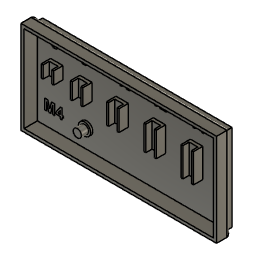
M4 Reference Caliper From 6 v4 (Autodesk Fusion 360 design; units mm, degrees)
Autodesk Fusion 360 part; units mm, degrees
note: some values were not read from the file. Chosen so that the rebuilt part matches the saved one: which bodies a step acts on; which pieces of a blend or face edit are solid.
sketch "Schizzo1" plane through (0, 0, 0) normal (0, 1, 0) x (1, 0, 0)
  line L0 (-43.0702, -47.1256) -> (51.9298, -47.1256)
  line L1 (51.9298, -47.1256) -> (51.9298, -2.1256)
  line L2 (51.9298, -2.1256) -> (-43.0702, -2.1256)
  line L3 (-43.0702, -2.1256) -> (-43.0702, -47.1256)
  line L4 (-34.9398, -37.9923) -> (-30.6504, -37.9923) construction
  line L5 (-30.6504, -37.9923) -> (-30.6504, -43.6096) construction
  line L6 (-30.6504, -43.6096) -> (-34.9398, -43.6096) construction
  line L7 (-34.9398, -43.6096) -> (-34.9398, -37.9923) construction
  line L8 (-20.4362, -37.9923) -> (-16.447, -37.9923) construction
  line L9 (-16.447, -37.9923) -> (-16.447, -43.6096) construction
  line L10 (-16.447, -43.6096) -> (-20.4362, -43.6096) construction
  line L11 (-20.4362, -43.6096) -> (-20.4362, -37.9923) construction
  line L12 (-2.7087, -37.9923) -> (2.1333, -37.9923) construction
  line L13 (2.1333, -37.9923) -> (2.1333, -43.6096) construction
  line L14 (2.1333, -43.6096) -> (-2.7087, -43.6096) construction
  line L15 (-2.7087, -43.6096) -> (-2.7087, -37.9923) construction
  line L16 (14.1885, -37.9923) -> (20.8281, -37.9923) construction
  line L17 (20.8281, -37.9923) -> (20.8281, -43.6096) construction
  line L18 (20.8281, -43.6096) -> (14.1885, -43.6096) construction
  line L19 (14.1885, -43.6096) -> (14.1885, -37.9923) construction
  line L20 (32.7115, -37.9923) -> (40.1532, -37.9923) construction
  line L21 (40.1532, -37.9923) -> (40.1532, -43.6096) construction
  line L22 (40.1532, -43.6096) -> (32.7115, -43.6096) construction
  line L23 (32.7115, -43.6096) -> (32.7115, -37.9923) construction
  line L24 (-35.1629, -33.0713) -> (-29.1629, -33.0713)
  line L25 (-29.1629, -33.0713) -> (-29.1629, -27.0713)
  line L26 (-29.1629, -27.0713) -> (-35.1629, -27.0713)
  line L27 (-35.1629, -27.0713) -> (-35.1629, -33.0713)
  line L28 (-32.1629, -33.0713) -> (-32.1629, -27.0713) construction
  line L29 (-30.0629, -27.0713) -> (-34.2629, -27.0713)
  line L30 (-34.2629, -27.0713) -> (-34.2629, -33.0713)
  line L31 (-34.2629, -33.0713) -> (-30.0629, -33.0713)
  line L32 (-30.0629, -33.0713) -> (-30.0629, -27.0713)
  line L33 (-30.0629, -27.0713) -> (-34.2629, -33.0713) construction
  line L34 (-34.2629, -27.0713) -> (-30.0629, -33.0713) construction
  line L35 (-14.9964, -25.0713) -> (-20.9964, -25.0713)
  line L36 (-20.0964, -25.0713) -> (-15.8964, -33.0713) construction
  line L37 (-15.8964, -25.0713) -> (-20.0964, -25.0713)
  line L38 (-15.8964, -33.0713) -> (-15.8964, -25.0713)
  line L39 (-20.0964, -25.0713) -> (-20.0964, -33.0713)
  line L40 (-15.8964, -25.0713) -> (-20.0964, -33.0713) construction
  line L41 (-17.9964, -33.0713) -> (-17.9964, -25.0713) construction
  line L42 (-20.9964, -33.0713) -> (-14.9964, -33.0713)
  line L43 (-20.9964, -25.0713) -> (-20.9964, -33.0713)
  line L44 (-14.9964, -33.0713) -> (-14.9964, -25.0713)
  line L45 (-20.0964, -33.0713) -> (-15.8964, -33.0713)
  line L46 (1.6974, -33.0713) -> (1.6974, -23.0713)
  line L47 (-3.4026, -23.0713) -> (-3.4026, -33.0713)
  line L48 (2.5974, -33.0713) -> (2.5974, -23.0713)
  line L49 (-3.4026, -33.0713) -> (2.5974, -33.0713)
  line L50 (1.6974, -23.0713) -> (-2.5026, -33.0713) construction
  line L51 (1.6974, -23.0713) -> (-2.5026, -23.0713)
  line L52 (-2.5026, -23.0713) -> (-2.5026, -33.0713)
  line L53 (-2.5026, -23.0713) -> (1.6974, -33.0713) construction
  line L54 (2.5974, -23.0713) -> (-3.4026, -23.0713)
  line L55 (-0.4026, -33.0713) -> (-0.4026, -23.0713) construction
  line L56 (-2.5026, -33.0713) -> (1.6974, -33.0713)
  line L57 (15.58, -33.0713) -> (19.78, -33.0713)
  line L58 (15.58, -21.0713) -> (15.58, -33.0713)
  line L59 (14.68, -33.0713) -> (20.68, -33.0713)
  line L60 (19.78, -33.0713) -> (19.78, -21.0713)
  line L61 (19.78, -21.0713) -> (15.58, -33.0713) construction
  line L62 (20.68, -21.0713) -> (14.68, -21.0713)
  line L63 (17.68, -33.0713) -> (17.68, -21.0713) construction
  line L64 (14.68, -21.0713) -> (14.68, -33.0713)
  line L65 (19.78, -21.0713) -> (15.58, -21.0713)
  line L66 (15.58, -21.0713) -> (19.78, -33.0713) construction
  line L67 (20.68, -33.0713) -> (20.68, -21.0713)
  line L68 (-43.0702, -33.0713) -> (51.9298, -33.0713) construction
  line L69 (32.7212, -33.0713) -> (38.7212, -33.0713)
  line L70 (37.8212, -19.0713) -> (33.6212, -33.0713) construction
  line L71 (38.7212, -33.0713) -> (38.7212, -19.0713)
  line L72 (32.7212, -19.0713) -> (32.7212, -33.0713)
  line L73 (37.8212, -33.0713) -> (37.8212, -19.0713)
  line L74 (37.8212, -19.0713) -> (33.6212, -19.0713)
  line L75 (35.7212, -33.0713) -> (35.7212, -19.0713) construction
  line L76 (33.6212, -19.0713) -> (33.6212, -33.0713)
  line L77 (33.6212, -33.0713) -> (37.8212, -33.0713)
  line L78 (33.6212, -19.0713) -> (37.8212, -33.0713) construction
  line L79 (38.7212, -19.0713) -> (32.7212, -19.0713)
  line L80 (-43.0702, -43.6096) -> (51.9298, -43.6096) construction
  line L81 (50.4298, -45.6256) -> (50.4298, -3.6256)
  line L82 (50.4298, -3.6256) -> (-41.5702, -3.6256)
  line L83 (-41.5702, -3.6256) -> (-41.5702, -45.6256)
  line L84 (-41.5702, -45.6256) -> (50.4298, -45.6256)
  line L85 (-38, -10) -> (-25, -10) construction
  line L86 (-25, -10) -> (-25, -15) construction
  line L87 (-25, -15) -> (-38, -15) construction
  line L88 (-38, -15) -> (-38, -10) construction
  line L89 (-43.0702, -37.9923) -> (50.4298, -37.9923) construction
  circle A0 centre (-17.6815, -12.6421) radius 2
  circle A1 centre (-17.6815, -12.6421) radius 3
  point P0 (-32.1629, -30.0713)
  point P1 (-17.9964, -29.0713)
  point P2 (-0.4026, -28.0713)
  point P3 (17.68, -27.0713)
  point P4 (35.7212, -26.0713)
  dimension "d1" = 45
  dimension "d2" = 5
  dimension "d3" = 5
  dimension "d4" = 5
  dimension "d5" = 5
  dimension "d6" = 5
  dimension "d7" = 6
  dimension "d8" = 6
  dimension "d9" = 4.2
  dimension "d21" = 6
  dimension "d22" = 8
  dimension "d23" = 4.2
  dimension "d24" = 6
  dimension "d25" = 10
  dimension "d26" = 4.2
  dimension "d27" = 6
  dimension "d28" = 12
  dimension "d29" = 4.2
  dimension "d30" = 6
  dimension "d31" = 14
  dimension "d32" = 4.2
  dimension "d33" = 95
  dimension "d34" = -1.5
  dimension "d37" = 5
  dimension "d40" = 4
  dimension "d41" = 6
  text T0 "6" font "Arial" height 5 bold align left middle in box 4.2894 x 5.6173 at (-34.9398, -37.9923) x (1, 0) y (0, -1) spacing 1
  text T1 "8" font "Arial" height 5 bold align left top in box 3.9891 x 5.6173 at (-20.4362, -37.9923) x (1, 0) y (0, -1) spacing 1
  text T2 "10\n" font "Arial" height 5 bold align left top in box 4.842 x 5.6173 at (-2.7087, -37.9923) x (1, 0) y (0, -1) spacing 1
  text T3 "12" font "Arial" height 5 bold align left top in box 6.6397 x 5.6173 at (14.1885, -37.9923) x (1, 0) y (0, -1) spacing 1
  text T4 "14" font "Arial" height 5 bold align left top in box 7.4417 x 5.6173 at (32.7115, -37.9923) x (1, 0) y (0, -1) spacing 1
  text T5 "M4" font "Arial" height 5 bold align left top in box 13 x 5 at (-38, -10) x (1, 0) y (0, -1) spacing 1
  constraint horizontal L0
  constraint vertical L1
  constraint horizontal L2
  constraint vertical L3
  constraint horizontal L24
  constraint vertical L25
  constraint horizontal L26
  constraint vertical L27
  constraint midpoint L24 L28.start
  constraint midpoint L26 L28.end
  constraint horizontal L29
  constraint perpendicular L29 L30
  constraint parallel L29 L31
  constraint parallel L30 L32
  constraint coincident L33 P0
  constraint coincident L34 P0
  constraint coincident L26 L29.start
  constraint midpoint L28 P0
  constraint horizontal L42
  constraint vertical L44
  constraint horizontal L35
  constraint vertical L43
  constraint midpoint L41.start L42
  constraint midpoint L41.end L35
  constraint horizontal L37
  constraint perpendicular L37 L39
  constraint parallel L37 L45
  constraint parallel L38 L39
  constraint coincident P1 L40
  constraint coincident P1 L36
  constraint coincident L37.start L35
  constraint midpoint P1 L41
  constraint horizontal L49
  constraint vertical L48
  constraint horizontal L54
  constraint vertical L47
  constraint midpoint L55.start L49
  constraint midpoint L55.end L54
  constraint horizontal L51
  constraint perpendicular L51 L52
  constraint parallel L51 L56
  constraint parallel L46 L52
  constraint coincident P2 L50
  constraint coincident P2 L53
  constraint coincident L46.end L54
  constraint midpoint P2 L55
  constraint horizontal L59
  constraint vertical L67
  constraint horizontal L62
  constraint vertical L64
  constraint midpoint L63.start L59
  constraint midpoint L63.end L62
  constraint horizontal L65
  constraint perpendicular L58 L65
  constraint parallel L57 L65
  constraint parallel L58 L60
  constraint coincident P3 L61
  constraint coincident P3 L66
  constraint coincident L60.end L62
  constraint midpoint P3 L63
  constraint coincident L3 L68.start
  constraint coincident L1 L68.end
  constraint perpendicular L1 L68
  constraint collinear L31 L68
  constraint collinear L49 L68
  constraint collinear L59 L68
  constraint horizontal L69
  constraint vertical L71
  constraint horizontal L79
  constraint vertical L72
  constraint midpoint L75.start L69
  constraint midpoint L75.end L79
  constraint horizontal L74
  constraint perpendicular L74 L76
  constraint parallel L74 L77
  constraint parallel L73 L76
  constraint coincident P4 L70
  constraint coincident P4 L78
  constraint coincident L70.start L79
  constraint midpoint P4 L75
  constraint coincident L3 L80.start
  constraint coincident L1 L80.end
  constraint perpendicular L1 L80
  constraint collinear L42 L68
  constraint collinear L68 L69
  constraint collinear L6 L80
  constraint collinear L10 L80
  constraint collinear L14 L80
  constraint collinear L18 L80
  constraint collinear L22 L80
  constraint coincident L3 L89.start
  constraint coincident L81 L89.end
  constraint perpendicular L81 L89
  constraint collinear L4 L89
  constraint collinear L8 L89
  constraint collinear L12 L89
  constraint collinear L16 L89
  constraint collinear L20 L89
  constraint concentric A0 A1
  measures "d1" distance of L0 L2
  measures "d7" distance of L24.start L24.end
  measures "d8" distance of L24.start L26.end
  measures "d9" distance of L30 L32
  measures "d21" distance of L42.start L42.end
  measures "d22" distance of L42.start L35.end
  measures "d23" distance of L38 L39
  measures "d24" distance of L47.end L48.start
  measures "d25" distance of L47.start L47.end
  measures "d26" distance of L46 L52
  measures "d27" distance of L59.end L59.start
  measures "d28" distance of L62.end L59.start
  measures "d29" distance of L58 L60
  measures "d30" distance of L69.start L69.end
  measures "d31" distance of L69.start L72.start
  measures "d32" distance of L73 L76
  measures "d33" distance of L1 L3
  measures "d40" diameter of A0
  measures "d41" diameter of A1
extrude "Estrusione1" add sketch "Schizzo1" along normal blind 0.4 text T0 T1 T2 T3 T4 T5 makes body 1 at (-34.2253, 0, 40.762) makes body 2 at (38.8382, 0, 42.0851) makes body 3 at (3.8192, 0, 40.7205) makes body 4 at (-18.3806, 0, 41.2901) makes body 5 at (19.2999, 0, 38.9063) makes body 6 at (34.5885, 0, 41.4871) makes body 7 at (-29.8815, 0, 13.4754) makes body 8 at (-37.6874, 0, 12.9786) makes body 9 at (-0.8317, 0, 41.4871) makes body 10 at (16.0655, 0, 41.4871)
extrude "Estrusione2" add sketch "Schizzo1" along normal blind 0.5 separate body contours L0 L1 L2 L3 | L24 L26 L27 L30 | L24 L26 L29 L30 L31 L32 | L24 L25 L26 L32 | L35 L38 L42 L44 | L35 L37 L38 L39 L42 L45 | L35 L39 L42 L43 | L46 L49 L51 L52 L54 L56 | L46 L48 L49 L54 | L47 L49 L52 L54 | L57 L58 L59 L60 L62 L65 | L58 L59 L62 L64 | L59 L60 L62 L67 | L69 L72 L76 L79 | L69 L73 L74 L76 L77 L79 | L69 L71 L73 L79 | L81 L82 L83 L84 | A0 | A1 makes body 11
extrude "Estrusione7" cut sketch "Schizzo1" along normal blind 0.4 text T0 T1 T2 T3 T5 T4 bodies 11
extrude "Estrusione6" add sketch "Schizzo1" against normal blind 6.5 contours L0 L1 L2 L3 bodies 11
extrude "Estrusione4" add sketch "Schizzo1" against normal blind 4.5 contours L24 L26 L27 L30 | L24 L26 L29 L30 L31 L32 | L24 L25 L26 L32 | L35 L38 L42 L44 | L35 L37 L38 L39 L42 L45 | L35 L39 L42 L43 | L46 L49 L51 L52 L54 L56 | L46 L48 L49 L54 | L47 L49 L52 L54 | L57 L58 L59 L60 L62 L65 | L58 L59 L62 L64 | L59 L60 L62 L67 | L69 L72 L76 L79 | L69 L73 L74 L76 L77 L79 | L69 L71 L73 L79 | A0 bodies 11
extrude "Estrusione8" add sketch "Schizzo1" against normal blind 1 contours A1 bodies 11
extrude "Estrusione5" cut sketch "Schizzo1" along normal blind 3 from surface at -4.5 contours L24 L26 L29 L30 L31 L32 | L35 L37 L38 L39 L42 L45 | L46 L49 L51 L52 L54 L56 | L57 L58 L59 L60 L62 L65 | L69 L73 L74 L76 L77 L79 bodies 11
sketch "Schizzo2" plane through (0, 0.5, 0) normal (0, 1, 0) x (-1, 0, 0)
  line L0 (43.0702, 2.1256) -> (43.0702, 47.1256)
  line L1 (43.0702, 47.1256) -> (-51.9298, 47.1256)
  line L2 (-51.9298, 47.1256) -> (-51.9298, 2.1256)
  line L3 (-51.9298, 2.1256) -> (43.0702, 2.1256)
  line L4 (-51.9298, 47.1256) -> (43.0702, 47.1256) construction
  line L5 (43.0702, 47.1256) -> (43.0702, 2.1256) construction
  line L6 (43.0702, 2.1256) -> (-51.9298, 2.1256) construction
  line L7 (-51.9298, 2.1256) -> (-51.9298, 47.1256) construction
  line L8 (-51.9298, 24.6256) -> (-50, 24.6256) construction
  line L9 (-50, 24.6256) -> (43.0702, 24.6256) construction
  line L10 (-4.4298, 47.1256) -> (-4.4298, 2.1256) construction
  line L11 (41.5702, 3.6256) -> (-50.4298, 3.6256)
  line L12 (-50.4298, 3.6256) -> (-50.4298, 45.6256)
  line L13 (-50.4298, 45.6256) -> (41.5702, 45.6256)
  line L14 (41.5702, 45.6256) -> (41.5702, 3.6256)
  line L15 (41.5702, 3.6256) -> (-50.4298, 45.6256) construction
  line L16 (-50.4298, 3.6256) -> (41.5702, 45.6256) construction
  point P0 (-4.4298, 24.6256)
  dimension "d44" = 1.5
  dimension "d45" = 1.5
  constraint horizontal L4
  constraint vertical L5
  constraint horizontal L6
  constraint vertical L7
  constraint coincident L0.end L1.start
  constraint coincident L2.end L3.start
  constraint midpoint L7 L8.start
  constraint perpendicular L7 L8
  constraint midpoint L5 L9.end
  constraint perpendicular L5 L9
  constraint midpoint L4 L10.start
  constraint midpoint L6 L10.end
  constraint horizontal L11
  constraint perpendicular L11 L12
  constraint parallel L11 L13
  constraint parallel L12 L14
  constraint coincident L15 P0
  constraint coincident L16 P0
  constraint midpoint L10 P0
  measures "d44" distance of L7 L12
  measures "d45" distance of L4 L13
extrude "Estrusione9" add sketch "Schizzo2" along normal blind 2 contours L11 L12 L13 L14 bodies 11
fillet "Raccordo1" radius 2 4 edges at (51.9298, 0.5, 24.6256) (4.4298, 0.5, 2.1256) (-43.0702, 0.5, 24.6256) (4.4298, 0.5, 47.1256) on bodies 11
equation "d21 = d7"
equation "d23 = d9"
equation "d24 = d7"
equation "d26 = d9"
equation "d27 = d7"
equation "d29 = d9"
equation "d30 = d7"
equation "d32 = d9"
equation "d41 = d40 + 2 mm"
equation "d45 = d44"
